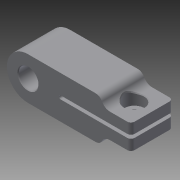
# Autodesk Inventor part: StringClamp
Saved by Autodesk Inventor 2015 (Build 190159000, 159)
## iProperties
Created: 2014-11-12
Part Number: StringClamp
Material: Generic
Document SubType Name: Modeling
Designer: Ryan
Density: 1 g/cm^3
Appearance: Default
Author: Ryan
Autodesk Inventor part; units mm, degrees
ref_plane "YZ Plane" through (0, 0, 0) normal (1, 0, 0) x (0, 1, 0)
ref_plane "XZ Plane" through (0, 0, 0) normal (0, 1, 0) x (-1, 0, 0)
ref_plane "XY Plane" through (0, 0, 0) normal (0, 0, 1) x (1, 0, 0)
sketch "Sketch1" plane through (0, 0, 0) normal (0, 0, 1) x (1, 0, 0)
  line L0 (0, 0) -> (0, 0.56) construction
  line L1 (0, 0) -> (-1.0158, 0) construction
  line L2 (-4.65, 3) -> (5.75, 3)
  line L3 (5.75, -3) -> (-4.65, -3)
  line L4 (10, 0.25) -> (0, 0.25)
  line L5 (10, -0.25) -> (0, -0.25)
  arc A0 (0, 0.25) -> (0, -0.25) centre (0, 0) ccw
  line L6 (10, 1.75) -> (7, 1.75)
  line L7 (10, -1.75) -> (7, -1.75)
  arc A1 (-4.65, 3) -> (-4.65, -3) centre (-4.65, 0) ccw
  circle A2 centre (-4.65, 0) radius 1.4
  line L8 (10, 1.75) -> (10, 0.25)
  line L9 (10, -0.25) -> (10, -1.75)
  arc A3 (5.75, 3) -> (7, 1.75) centre (7, 3) ccw
  arc A4 (7, -1.75) -> (5.75, -3) centre (7, -3) ccw
  dimension "d2" = 0.5
  dimension "d5" = 2.8
  dimension "d6" = 6
  dimension "d8" = 10
  dimension "d9" = 1.5
  dimension "d10" = 3
  dimension "d12" = 3
  constraints: 20 end point, 8 point on circle, 6 tangent, 5 centre point, 5 horizontal, 2 coincident, 2 perpendicular, 1 collinear, 1 line through centre, 1 parallel, 1 point on line, 1 vertical, 1 vertical alignment, 5 other
  measures "d2" distance between parallel lines of L5 L4
  measures "d5" diameter of A2
  measures "d6" distance between parallel lines of L3 L2
  measures "d8" distance of L4.start L4.end
  measures "d9" distance of L5.start L7.start
  measures "d10" distance of L6.start L6.end
extrude "Extrusion1" add sketch "Sketch1" along normal blind 6
sketch "Sketch2" plane through (7, 1.75, 0) normal (0, 1, 0) x (1, 0, 0)
  circle A0 centre (0.5, -3.0099) radius 1.4
  line L0 (3, 0) -> (3, -6) projected
  point P0 (-7, 0)
  dimension "d15" = 2.8
  dimension "d16" = 2.5
  constraints: 1 centre point
  measures "d15" diameter of A0
  measures "d16" distance from line of L0 A0.centre
extrude "Extrusion2" cut sketch "Sketch2" along normal through all both and the other way through all
fillet "Fillet1" radius 0.5 1 edges at (10, 1, 6)
fillet "Fillet2" radius 0.5 1 edges at (10, -1, 6)
fillet "Fillet3" radius 0.5 1 edges at (10, 1, 0)
fillet "Fillet4" radius 0.5 1 edges at (10, -1, 0)
fillet "Fillet5" radius 1 1 edges at (5.75, 3, 3)
fillet "Fillet6" radius 1 1 edges at (5.75, -3, 3)
chamfer "Chamfer1" distance 0.1 angle 45 1 edges at (-6.05, 0, 6)
chamfer "Chamfer2" distance 0.1 angle 45 3 edges at (6.1, 2.1325, 3.0079) (8.2937, 1.75, 1.8567) (8.2937, 1.75, 4.1632)
equation "\"d17\" = d15"
body "Solid1"
